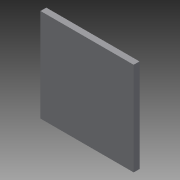
# Autodesk Inventor part: fai6_sikiita
Saved by Autodesk Inventor 2013 (Build 170138000, 138)
## iProperties
Created: 2014-04-21
Part Number: fai6_sikiita
Material: 一般
Document SubType Name: Modeling
Designer: andou
Density: 1 g/cm^3
Author: andou
Autodesk Inventor part; units mm, degrees
ref_plane "YZ Plane" through (0, 0, 0) normal (1, 0, 0) x (0, 1, 0)
ref_plane "XZ Plane" through (0, 0, 0) normal (0, 1, 0) x (-1, 0, 0)
ref_plane "XY Plane" through (0, 0, 0) normal (0, 0, 1) x (1, 0, 0)
sketch "スケッチ1" plane through (0, 0, 0) normal (0, 1, 0) x (-1, 0, 0)
  line L0 (-20, 20) -> (20, 20)
  line L1 (20, 20) -> (20, -20)
  line L2 (20, -20) -> (-20, -20)
  line L3 (-20, -20) -> (-20, 20)
  point P0 (0, 0)
  dimension "d0" = 40
  dimension "d2" = 40
  dimension "d3" = 20
  dimension "d4" = 20
  constraints: 8 end point, 2 parallel, 1 horizontal, 1 perpendicular
  measures "d0" distance of L0.start L0.end
  measures "d2" distance of L2.end L0.start
  measures "d3" distance from line of L2 point (0, 0)
  measures "d4" distance from line of L1 point (0, 0)
extrude "押し出し1" add sketch "スケッチ1" along normal blind 2
sketch "スケッチ2" plane through (0, 2, 0) normal (0, 1, 0) x (1, 0, 0)
  line L0 (-20, -20) -> (20, -20) projected
  line L1 (20, -20) -> (20, 20) projected
  line L2 (20, 20) -> (-20, 20) projected
  line L3 (-20, 20) -> (-20, -20) projected
  circle A0 centre (-15, -15) radius 3
  circle A1 centre (-5, -15) radius 3
  circle A2 centre (5, -15) radius 3
  circle A3 centre (15, -15) radius 3
  circle A4 centre (-15, -5) radius 3
  circle A5 centre (-15, 5) radius 3
  circle A6 centre (-15, 15) radius 3
  circle A7 centre (-5, -5) radius 3
  circle A8 centre (-5, 5) radius 3
  circle A9 centre (-5, 15) radius 3
  circle A10 centre (5, -5) radius 3
  circle A11 centre (15, -5) radius 3
  circle A12 centre (15, 5) radius 3
  circle A13 centre (5, 5) radius 3
  circle A14 centre (5, 15) radius 3
  circle A15 centre (15, 15) radius 3
  point P0 (0, 0)
  dimension "d7" = 6
  dimension "d9" = 10
  dimension "d10" = 10
  dimension "d11" = 10
  dimension "d12" = 5
  dimension "d13" = 5
  dimension "d14" = 5
  dimension "d15" = 5
  dimension "d16" = 5
  dimension "d17" = 10
  dimension "d18" = 10
  dimension "d19" = 10
  dimension "d20" = 5
  dimension "d21" = 5
  dimension "d22" = 5
  dimension "d23" = 10
  dimension "d24" = 10
  dimension "d25" = 10
  dimension "d26" = 10
  dimension "d27" = 10
  dimension "d28" = 10
  dimension "d29" = 10
  dimension "d30" = 10
  dimension "d31" = 10
  dimension "d32" = 10
  dimension "d33" = 10
  dimension "d34" = 10
  dimension "d35" = 10
  dimension "d36" = 10
  dimension "d37" = 10
  dimension "d38" = 10
  dimension "d39" = 10
  dimension "d40" = 10
  constraints: 16 centre point, 15 equal radius
  measures "d7" diameter of A0
  measures "d9" distance of A1.centre A0.centre
  measures "d10" distance of A2.centre A1.centre
  measures "d11" distance of A3.centre A2.centre
  measures "d12" distance from line of A0.centre L0
  measures "d13" distance from line of L3 A0.centre
  measures "d14" distance from line of L0 A1.centre
  measures "d15" distance from line of L0 A2.centre
  measures "d16" distance from line of L0 A3.centre
  measures "d17" distance of A4.centre A0.centre
  measures "d18" distance of A4.centre A5.centre
  measures "d19" distance of A5.centre A6.centre
  measures "d20" distance from line of L3 A4.centre
  measures "d21" distance from line of L3 A5.centre
  measures "d22" distance from line of L3 A6.centre
  measures "d23" distance of A4.centre A7.centre
  measures "d24" distance of A7.centre A1.centre
  measures "d25" distance of A2.centre A10.centre
  measures "d26" distance of A11.centre A3.centre
  measures "d27" distance of A11.centre A10.centre
  measures "d28" distance of A7.centre A10.centre
  measures "d29" distance of A8.centre A13.centre
  measures "d30" distance of A9.centre A14.centre
  measures "d31" distance of A9.centre A8.centre
  measures "d32" distance of A14.centre A13.centre
  measures "d33" distance of A13.centre A12.centre
  measures "d34" distance of A14.centre A15.centre
  measures "d35" distance of A15.centre A12.centre
  measures "d36" distance of A6.centre A9.centre
  measures "d37" distance of A5.centre A8.centre
  measures "d38" distance of A8.centre A7.centre
  measures "d39" distance of A13.centre A10.centre
  measures "d40" distance of A12.centre A11.centre
extrude "押し出し2" add sketch "スケッチ2" along normal blind 0.5
